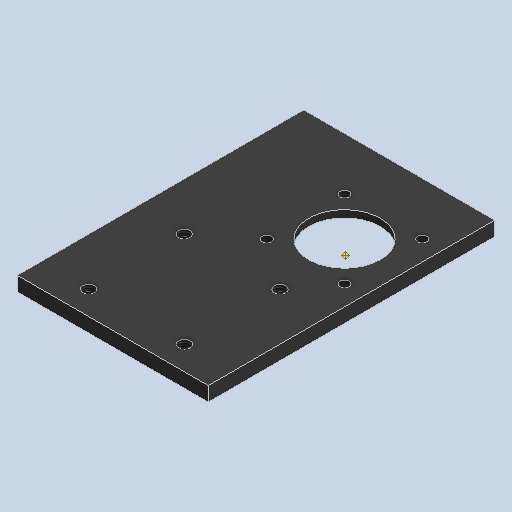
# Autodesk Inventor part: Platform
Saved by Autodesk Inventor 2023 (Build 270158000, 158)
## iProperties
Created: 2022-01-09
Part Number: Platform
Material: Generico
Document SubType Name: Sheet Metal
Designer: Elia
Density: 1 g/cm^3
Sheet Metal Rule: Default_mm
Appearance: Gomma - Nero
Author: Elia
Autodesk Inventor part; units mm, degrees
ref_plane "YZ Plane" through (0, 0, 0) normal (1, 0, 0) x (0, 1, 0)
ref_plane "XZ Plane" through (0, 0, 0) normal (0, 1, 0) x (-1, 0, 0)
ref_plane "XY Plane" through (0, 0, 0) normal (0, 0, 1) x (1, 0, 0)
sketch "Schizzo1" plane through (0, 0, 0) normal (0, 1, 0) x (-1, 0, 0)
  line L0 (87.6536, 7.4302) -> (-32.3464, 7.4302)
  line L1 (-32.3464, 7.4302) -> (-32.3464, -72.5698)
  line L2 (-32.3464, -72.5698) -> (87.6536, -72.5698)
  line L3 (87.6536, -72.5698) -> (87.6536, 7.4302)
  point P0 (0, 0)
  dimension "d0" = 80
  dimension "d1" = 120
  constraints: 8 end point, 2 parallel, 1 horizontal, 1 perpendicular
  measures "d0" distance between parallel lines of L2 L0
  measures "d1" distance between parallel lines of L1 L3
extrude "Estrusione1" add sketch "Schizzo1" along normal blind 6
move or copy body "Sposta corpo1" bodies to move or copy 1 copy no rotation origin (0, 0, 0) rotation axis (0, 1, 0) rotation angle 90 translate (9.9162, 0, -65.2235)
sketch "Schizzo7" plane through (-62.6536, 0, -97.5698) normal (0, -1, 0) x (1, 0, 0)
  circle A0 centre (19.9435, 110) radius 4
  circle A1 centre (19.9435, 70) radius 4
  circle A2 centre (60.0565, 70) radius 4
  circle A3 centre (60.0565, 110) radius 4
  constraints: 4 centre point, 8 other
hole "Foro1" at (-2.5971, 0, 12.4302) at (-2.5971, 0, -27.5698) at (-42.7101, 0, -27.5698) at (-42.7101, 0, 12.4302) direction (0, 1, 0) diameter 4.917 end through all counterbore diameter 10.5 counterbore depth 3.3 thread size "M6x1" class "6H" standard "ANSI Metric M Profile"
sketch "Schizzo8" plane through (-62.6536, 0, -97.5698) normal (0, -1, 0) x (1, 0, 0)
  line L0 (75.3545, 58.287) -> (35.3545, 58.287)
  line L1 (35.3545, 58.287) -> (35.3545, 18.287)
  line L2 (35.3545, 18.287) -> (75.3545, 18.287)
  line L3 (75.3545, 18.287) -> (75.3545, 58.287)
  circle A0 centre (55.3545, 38.287) radius 15
  circle A1 centre (39.0911, 54.5505) radius 2.25
  circle A2 centre (71.618, 54.5505) radius 2.25
  circle A3 centre (39.0911, 22.0236) radius 2.25
  circle A4 centre (71.618, 22.0236) radius 2.25
  point P0 (62.6536, 97.5698)
  dimension "d14" = 30
  dimension "d16" = 4.5
  dimension "d17" = 4.5
  dimension "d18" = 4.5
  dimension "d19" = 4.5
  constraints: 8 end point, 5 centre point, 5 coincident, 2 parallel, 1 horizontal, 1 perpendicular
  measures "d14" diameter of A0
  measures "d16" diameter of A1
  measures "d17" diameter of A2
  measures "d18" diameter of A3
  measures "d19" diameter of A4
hole "Foro2" at (8.9643, 0, -43.0193) direction (0, 1, 0) diameter 3.9587 depth 6 thread size "M4.5x0.5" class "6H" standard "ANSI Metric M Profile"
hole "Foro3" at (-23.5626, 0, -43.0193) direction (0, 1, 0) diameter 3.9587 depth 6 thread size "M4.5x0.5" class "6H" standard "ANSI Metric M Profile"
hole "Foro4" at (-23.5626, 0, -75.5463) direction (0, 1, 0) diameter 3.9587 depth 6 thread size "M4.5x0.5" class "6H" standard "ANSI Metric M Profile"
hole "Foro5" at (8.9643, 0, -75.5463) direction (0, 1, 0) diameter 3.9587 depth 6 thread size "M4.5x0.5" class "6H" standard "ANSI Metric M Profile"
sketch "Schizzo9" plane through (-62.6536, 0, -97.5698) normal (0, -1, 0) x (1, 0, 0)
  line L0 (35.3545, 58.287) -> (75.3545, 58.287)
  line L1 (75.3545, 58.287) -> (75.3545, 18.287)
  line L2 (75.3545, 18.287) -> (35.3545, 18.287)
  line L3 (35.3545, 18.287) -> (35.3545, 58.287)
  point P0 (62.6536, 97.5698)
  point P1 (35.3545, 18.287)
  point P2 (75.3545, 58.287)
  point P3 (55.3545, 38.287)
  constraints: 8 end point, 2 parallel, 1 horizontal, 1 perpendicular, 1 other
extrude "Estrusione2" cut sketch "Schizzo9" against normal blind 3
hole "Foro6" at (-7.2991, 0, -59.2828) direction (0, 1, 0) diameter 30 depth 6
equation "\"RaggioPiega\" = Spessore"
equation "\"LarghezzaScaricoPiega\" = Spessore"
equation "\"ProfonditàScaricoPiega\" = 0.5 * Spessore"
equation "\"DimensioniScaricoAngolo\" = 4 * Spessore"
equation "\"ResiduoMinimo\" = 2 * Spessore"
equation "\"RaggioTransizione\" = RaggioPiega"
equation "\"Dimensione_raggio_Jacobi\" = RaggioPiega"
equation "\"DimensioneGioco\" = Spessore"
equation "\"Spessore\" = 0.5"
